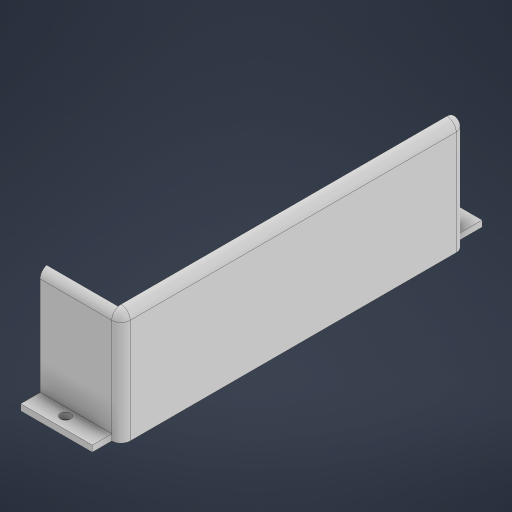
# Autodesk Inventor part: batre
Saved by Autodesk Inventor 2024.3 (Build 283343000, 343)
## iProperties
Created: 2025-06-23
Part Number: batre
Material: Generic
Document SubType Name: Modeling
Designer: Akbar Syihabuddin
Density: 1 g/cm^3
Appearance: Default
Author: Akbar Syihabuddin
Autodesk Inventor part; units mm, degrees
ref_plane "YZ Plane" through (0, 0, 0) normal (1, 0, 0) x (0, 1, 0)
ref_plane "XZ Plane" through (0, 0, 0) normal (0, 1, 0) x (-1, 0, 0)
ref_plane "XY Plane" through (0, 0, 0) normal (0, 0, 1) x (1, 0, 0)
sketch "Sketch1" plane through (0, 0, 0) normal (0, 1, 0) x (-1, 0, 0)
  line L0 (-1.6796, 1.0424) -> (10.8204, 1.0424)
  line L1 (10.8204, 1.0424) -> (10.8204, -53.9576)
  line L2 (10.8204, -53.9576) -> (-1.6796, -53.9576)
  line L3 (-1.6796, -53.9576) -> (-1.6796, 1.0424)
  line L4 (-1.6796, 1.0424) -> (-14.1796, 1.0424)
  line L5 (-14.1796, 1.0424) -> (-14.1796, -53.9576)
  line L6 (-14.1796, -53.9576) -> (-1.6796, -53.9576)
  line L7 (10.8204, 1.0424) -> (10.8204, 56.0424)
  line L8 (10.8204, 56.0424) -> (-1.6796, 56.0424)
  line L9 (-1.6796, 56.0424) -> (-1.6796, 1.0424)
  line L10 (-14.1796, 1.0424) -> (-14.1796, 56.0424)
  line L11 (-14.1796, 56.0424) -> (-1.6796, 56.0424)
  line L12 (10.8204, 56.0424) -> (-14.1796, 56.0424)
  line L13 (-14.1796, 56.0424) -> (-14.1796, 64.4726)
  line L14 (-14.1796, 64.4726) -> (10.8204, 64.4726)
  line L15 (10.8204, 64.4726) -> (10.8204, 56.0424)
  line L16 (10.8204, -53.9576) -> (-1.6796, -53.9576)
  line L17 (-14.1796, -53.9576) -> (-1.6796, -53.9576)
  line L18 (10.8204, -53.9576) -> (-14.1796, -53.9576)
  line L19 (10.8204, -62.3878) -> (10.8204, -53.9576)
  line L20 (-14.1796, -62.3878) -> (10.8204, -62.3878)
  line L21 (-14.1796, -53.9576) -> (-14.1796, -62.3878)
  line L22 (-1.6796, 56.0424) -> (-1.6796, 60.6584)
  circle A0 centre (-1.6796, 60.6584) radius 1.65
  circle A1 centre (-1.6796, -58.5736) radius 1.65
  point P0 (0, 0)
  point P1 (-14.6796, 1.0424)
  dimension "d0" = 12.5
  dimension "d1" = 55
  dimension "d2" = 4.616
  dimension "d3" = 3.3
  constraints: 46 end point, 4 parallel, 4 symmetric about line, 2 centre point, 2 coincident, 2 horizontal, 2 perpendicular, 1 vertical, 1 other
  measures "d0" distance of L1.end L3.start
  measures "d1" distance of L0.end L1.end
  measures "d2" distance of L9.start L22.end
  measures "d3" diameter of A0
extrude "Extrusion1" add sketch "Sketch1" along normal blind 2 contours L2 L19 L20 L21 L6 | L11 L13 L14 L15 L8 | A1
extrude "Extrusion2" add sketch "Sketch1" along normal blind 2 contours L9 L8 L7 L0 | L0 L1 L2 L3 | L3 L6 L5 L4 | L4 L10 L11 L9
sketch "Sketch3" plane through (14.1796, 0, 64.4726) normal (1, 0, 0) x (0, 0, -1)
  line L0 (0, 0) -> (126.8603, 0) projected
  line L1 (0, 2) -> (126.8603, 2) projected
  line L2 (63.4302, 0) -> (8.4302, 0)
  line L3 (8.4302, 0) -> (8.4302, 2)
  line L4 (8.4302, 2) -> (63.4302, 2)
  line L5 (63.4302, 2) -> (63.4302, 0)
  line L6 (63.4302, 2) -> (118.4302, 2)
  line L7 (118.4302, 2) -> (118.4302, 0)
  line L8 (118.4302, 0) -> (63.4302, 0)
  line L9 (63.4302, 0) -> (63.4302, 2)
  point P0 (64.4726, 0)
  dimension "d12" = 55
  dimension "d13" = 55
  constraints: 16 end point, 4 parallel, 2 horizontal, 2 perpendicular, 2 point on line, 1 midpoint
  measures "d12" distance of L3.end L4.end
  measures "d13" distance of L7.end L8.end
extrude "Extrusion4" add sketch "Sketch3" along normal blind 3
sketch "Sketch4" plane through (0, 2, 0) normal (0, 1, 0) x (1, 0, 0)
  line L0 (14.1796, -56.0424) -> (17.1796, -56.0424) projected
  line L1 (14.1796, 53.9576) -> (17.1796, 53.9576)
  line L2 (17.1796, 53.9576) -> (17.1796, -56.0424)
  line L3 (17.1796, -56.0424) -> (14.1796, -56.0424)
  line L4 (14.1796, -56.0424) -> (14.1796, 53.9576)
  point P0 (0, 0)
  constraints: 8 end point, 2 parallel, 1 horizontal, 1 perpendicular
extrude "Extrusion5" add sketch "Sketch4" along normal blind 35
sketch "Sketch5" plane through (-10.8204, 0, -62.3878) normal (-1, 0, 0) x (0, 0, 1)
  line L0 (0, 2) -> (126.8603, 2) projected
  line L1 (0, 2) -> (126.8603, 2)
  line L2 (126.8603, 2) -> (126.8603, 0)
  line L3 (126.8603, 0) -> (0, 0)
  line L4 (0, 0) -> (0, 2)
  point P0 (62.3878, 0)
  constraints: 8 end point, 2 parallel, 1 horizontal, 1 perpendicular
extrude "Extrusion6" add sketch "Sketch5" along normal blind 0.7
sketch "Sketch6" plane through (0, 2, 0) normal (0, 1, 0) x (1, 0, 0)
  line L0 (-11.5204, -64.4726) -> (-11.5204, 62.3878) projected
  line L1 (14.1796, -56.0424) -> (-11.5204, -56.0424)
  line L2 (-11.5204, -56.0424) -> (-11.5204, -58.1521)
  line L3 (-11.5204, -58.1521) -> (14.1796, -58.1521)
  line L4 (14.1796, -58.1521) -> (14.1796, -56.0424)
  point P0 (0, 0)
  point P1 (-11.5204, -56.0424)
  constraints: 8 end point, 2 parallel, 1 horizontal, 1 perpendicular, 1 point on line
extrude "Extrusion7" add sketch "Sketch6" along normal blind 35
sketch "Sketch7" plane through (14.1796, 0, 56.0424) normal (0, 0, 1) x (1, 0, 0)
  line L0 (0, 0) -> (0, 2) projected
  line L1 (3, 0) -> (3, 37) projected
  line L2 (0, 0) -> (3, 0)
  line L3 (3, 0) -> (3, 37)
  line L4 (3, 37) -> (0, 37)
  line L5 (0, 37) -> (0, 0)
  point P0 (-14.1796, 0)
  constraints: 8 end point, 2 parallel, 1 horizontal, 1 perpendicular
extrude "Extrusion8" add sketch "Sketch7" along normal blind 2.1
fillet "Fillet1" radius 3 1 edges at (17.1796, 18.5, 58.1424)
sketch "Sketch8" plane through (0, 2, 0) normal (0, 1, 0) x (1, 0, 0)
  circle A0 centre (1.6796, -60.6584) radius 1.65 projected
  circle A1 centre (1.6796, -60.6584) radius 1.65
  line L0 (-11.5204, 62.3878) -> (-11.5204, -64.4726) projected
  line L1 (-11.5204, -1.0424) -> (1.6796, -1.0424)
  circle A2 centre (1.6796, 58.5736) radius 1.65
  circle A3 centre (1.6796, 58.5736) radius 1.65
  point P0 (0, 0)
  constraints: 3 centre point, 2 coincident, 2 end point, 2 symmetric about line, 1 horizontal, 1 midpoint, 2 other
extrude "Extrusion9" cut sketch "Sketch8" against normal blind 2.1 contours A2
sketch "Sketch9" plane through (14.1796, 2, 56.0424) normal (0, 0, -1) x (-1, 0, 0)
  line L0 (0, 0) -> (0, 35) projected
  line L1 (0, 17.5) -> (23.3, 17.5)
  line L2 (25.7, 35) -> (0, 35) projected
  line L3 (23.3, 17.5) -> (25.7, 17.5)
  line L4 (25.7, 17.5) -> (25.7, 35)
  line L5 (25.7, 35) -> (23.3, 35)
  line L6 (23.3, 35) -> (23.3, 17.5)
  line L7 (23.3, 17.5) -> (25.7, 17.5)
  line L8 (25.7, 17.5) -> (25.7, -2)
  line L9 (25.7, -2) -> (23.3, -2)
  line L10 (23.3, -2) -> (23.3, 17.5)
  point P0 (14.1796, -2)
  dimension "d27" = 23.3
  constraints: 18 end point, 4 parallel, 3 horizontal, 2 perpendicular, 1 midpoint, 1 point on line
  measures "d27" distance of L1.start L1.end
extrude "Extrusion10" cut sketch "Sketch9" along normal mid plane 300 contours L6 L2 L4 L3 | L3 L8 L9 L10
fillet "Fillet2" radius 3 1 edges at (17.1796, 18.5, -53.9576)
fillet "Fillet3" radius 3 6 edges at (16.3009, 37, 57.2638) (14.1796, 37, 58.1424) (14.1796, 37, -53.9576) (16.3009, 37, -53.0789) (17.1796, 37, 2.0924) (2.5296, 37, 58.1521)
body "Solid1"
